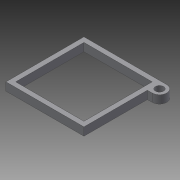
# Autodesk Inventor part: Stepper_Motor_Holder-SquareBar-Rev3
Saved by Autodesk Inventor 2015 (Build 190159000, 159)
## iProperties
Created: 2017-01-12
Part Number: Stepper_Motor_Holder-SquareBar-Rev3
Material: Generic
Document SubType Name: Modeling
Designer: Guy
Density: 1 g/cm^3
Appearance: Default
Author: Guy
Autodesk Inventor part; units mm, degrees
ref_plane "YZ Plane" through (0, 0, 0) normal (1, 0, 0) x (0, 1, 0)
ref_plane "XZ Plane" through (0, 0, 0) normal (0, 1, 0) x (-1, 0, 0)
ref_plane "XY Plane" through (0, 0, 0) normal (0, 0, 1) x (1, 0, 0)
sketch "Sketch1" plane through (0, 0, 0) normal (0, 0, 1) x (1, 0, 0)
  line L0 (0, 0) -> (42.3, 0)
  line L1 (42.3, 0) -> (42.3, 42.3)
  line L2 (42.3, 42.3) -> (0, 42.3)
  line L3 (0, 42.3) -> (0, 0)
  line L4 (45.3, -3) -> (45.3, 45.3)
  line L5 (-3, 45.3) -> (-3, -3)
  line L6 (-3, -3) -> (45.3, -3)
  circle A0 centre (39.3, 3) radius 1.5
  circle A1 centre (3, 3) radius 1.5
  circle A2 centre (3, 39.3) radius 1.5
  arc A3 (3, 36.3) -> (6, 39.3) centre (3, 39.3) ccw
  arc A4 (39.3, 6) -> (36.3, 3) centre (39.3, 3) ccw
  arc A5 (6, 3) -> (3, 6) centre (3, 3) ccw
  line L7 (0, 36.3) -> (3, 36.3)
  line L8 (6, 39.3) -> (6, 42.3)
  line L9 (42.3, 6) -> (39.3, 6)
  line L10 (36.3, 3) -> (36.3, 0)
  line L11 (6, 0) -> (6, 3)
  line L12 (3, 6) -> (0, 6)
  line L13 (-3, 45.3) -> (48.3, 45.3)
  circle A6 centre (48.3, 40.8) radius 2.5
  arc A7 (48.3, 36.3) -> (48.3, 45.3) centre (48.3, 40.8) ccw
  line L14 (45.3, 36.3) -> (48.3, 36.3)
  point P0 (45.3, 42.3)
  point P1 (45.3, 0)
  point P2 (-3, 0)
  point P3 (-3, 42.3)
  dimension "d0" = 42.3
  dimension "d1" = 42.3
  dimension "d3" = 3
  dimension "d5" = 3
  dimension "d29" = 3
  dimension "d30" = 3
  dimension "d31" = 3
  dimension "d32" = 3
  dimension "d34" = 3
  dimension "d35" = 3
  dimension "d38" = 3
  dimension "d39" = 3
  dimension "d40" = 3
  dimension "d41" = 3
  dimension "d43" = 3
  dimension "d50" = 5
  dimension "d51" = 9
  dimension "d52" = 3
  constraints: 30 end point, 12 point on line, 11 tangent, 8 centre point, 8 point on circle, 7 parallel, 4 coincident, 4 horizontal, 3 perpendicular
  measures "d0" distance of L0.end L1.end
  measures "d1" distance of L1.end L2.end
  measures "d3" distance between parallel lines of L4 L1
  measures "d5" distance between parallel lines of L3 L5
  measures "d29" distance between parallel lines of L6 L0
  measures "d30" diameter of A0
  measures "d31" diameter of A1
  measures "d32" diameter of A2
  measures "d34" distance from line of A2.centre L2
  measures "d35" distance from line of L3 A2.centre
  measures "d38" distance from line of L1 A0.centre
  measures "d39" distance from line of L0 A0.centre
  measures "d40" distance from line of L0 A1.centre
  measures "d41" distance from line of L3 A1.centre
  measures "d43" distance between parallel lines of L2 L13
  measures "d50" diameter of A6
  measures "d51" diameter of A7
  measures "d52" distance from line of L4 A7.centre
extrude "Extrusion6" add sketch "Sketch1" along normal blind 5 contours L6 L5 L13 L4 | L4 L13 A7 L14
body "Solid5"
